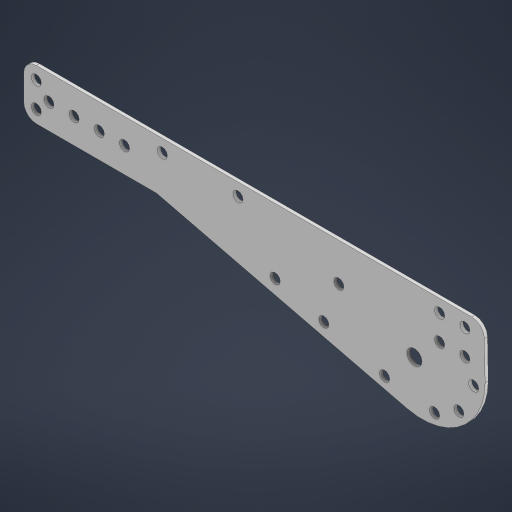
# Autodesk Inventor part: intake sled v5
Saved by Autodesk Inventor 2023.4 (Build 274418000, 418)
## iProperties
Created: 2023-12-16
Part Number: intake sled v5
Material: Generic
Document SubType Name: Modeling
Designer: Meer
Density: 1 g/cm^3
Appearance: Default
Author: Meer
Autodesk Inventor part; units mm, degrees
ref_plane "YZ Plane" through (0, 0, 0) normal (1, 0, 0) x (0, 1, 0)
ref_plane "XZ Plane" through (0, 0, 0) normal (0, 1, 0) x (-1, 0, 0)
ref_plane "XY Plane" through (0, 0, 0) normal (0, 0, 1) x (1, 0, 0)
sketch "Sketch1" plane through (0, 0, 0) normal (0, 0, 1) x (1, 0, 0)
  line L0 (0, 0) -> (247.65, 0)
  line L1 (247.65, 0) -> (247.65, 38.1)
  line L2 (247.65, 38.1) -> (0, 38.1)
  line L3 (0, 38.1) -> (0, 0)
  line L4 (286.1616, 0) -> (255.1962, 0)
  line L5 (255.1962, 0) -> (255.1962, 12.7)
  line L6 (255.1962, 12.7) -> (286.1616, 12.7)
  line L7 (286.1616, 12.7) -> (286.1616, 0)
  line L8 (247.65, 12.7) -> (200.66, 12.7)
  line L9 (16.2468, 38.1) -> (16.2468, 12.7)
  line L10 (16.2468, 12.7) -> (196.85, 12.7)
  line L11 (0, 12.7) -> (17.7951, 12.7)
  circle A0 centre (200.66, 12.7) radius 31.75
  line L12 (232.41, 12.7) -> (231.9451, 38.1)
  line L13 (66.8614, 12.7) -> (200.8653, -20.0324)
  line L14 (193.3963, -18.208) -> (168.91, 12.7)
  point P0 (187.853, -16.3524)
  point P1 (232.3887, 13.8619)
  point P2 (229.7594, 0)
  point P3 (181.61, 38.1)
  point P4 (219.71, 38.1)
  point P5 (171.5606, 0)
  dimension "d0" = 247.65
  dimension "d1" = 38.1
  dimension "d2" = 12.7
  dimension "d3" = 30.9654
  dimension "d4" = 46.99
  dimension "d10" = 25.4
  dimension "d54" = 63.5
  constraints: 30 end point, 10 point on line, 5 perpendicular, 4 parallel, 4 point on circle, 2 horizontal, 1 centre point, 1 coincident
  measures "d0" distance of L1.end L2.end
  measures "d1" distance of L0.end L1.end
  measures "d2" distance of L6.end L4.start
  measures "d3" distance of L5.end L6.end
  measures "d4" distance of L8.start L8.end
  measures "d10" distance of L9.start L9.end
  measures "d54" diameter of A0
extrude "Extrusion4" add sketch "Sketch1" along normal blind 1.5875 contours L13 L0 A0 | L13 L10 A0 L0 | L3 L2 L9 L11 | A0 L14 L0 | L0 L14 A0 | L10 L9 L2 A0 | L14 L0 A0 | L14 A0 L2 L12 L0 | L2 L12 A0
fillet "Fillet6" radius 6.35 3 edges at (0, 38.1, 0.7937) (0, 12.7, 0.7937) (231.9451, 38.1, 0.7937)
sketch "Sketch4" plane through (0, 0, 1.5875) normal (0, 0, 1) x (1, 0, 0)
  arc A0 (6.35, 38.1) -> (0, 31.75) centre (6.35, 31.75) ccw projected
  line L0 (6.35, 38.1) -> (6.35, 31.75)
  line L1 (6.35, 31.75) -> (0, 31.75)
  circle A1 centre (6.35, 31.75) radius 2.54
  line L2 (6.35, 31.75) -> (6.35, 19.05)
  circle A2 centre (6.35, 19.05) radius 2.54
  line L3 (6.35, 31.75) -> (57.15, 31.75)
  line L4 (57.15, 31.75) -> (107.95, 31.75)
  line L5 (107.95, 31.75) -> (158.75, 31.75)
  line L6 (158.75, 31.75) -> (209.55, 31.75)
  circle A3 centre (107.95, 31.75) radius 2.54
  circle A4 centre (209.55, 31.75) radius 2.54
  line L7 (57.15, 31.75) -> (57.15, 19.05)
  line L8 (57.15, 19.05) -> (107.95, 19.05)
  line L9 (107.95, 19.05) -> (158.75, 19.05)
  line L10 (158.75, 19.05) -> (209.55, 19.05)
  circle A5 centre (158.75, 19.05) radius 2.54
  circle A6 centre (209.55, 19.05) radius 2.54
  line L11 (225.7103, 38.1) -> (6.35, 38.1) projected
  arc A7 (193.3963, -18.208) -> (232.41, 12.7) centre (200.66, 12.7) ccw projected
  line L12 (209.55, 31.75) -> (196.85, 31.75)
  line L13 (196.85, 31.75) -> (196.85, 19.05)
  circle A8 centre (196.85, 31.75) radius 2.54
  line L14 (196.85, 19.05) -> (196.85, 6.096)
  circle A9 centre (196.85, 6.096) radius 3.81
  line L15 (57.15, 31.75) -> (69.85, 31.75)
  circle A10 centre (69.85, 31.75) radius 2.54
  point P0 (0, 0)
  point P1 (207.01, 31.75)
  dimension "d60" = 6.35
  dimension "d61" = 5.08
  dimension "d62" = 12.7
  dimension "d63" = 5.08
  dimension "d64" = 50.8
  dimension "d65" = 50.8
  dimension "d66" = 50.8
  dimension "d67" = 50.8
  dimension "d70" = 5.08
  dimension "d72" = 5.08
  dimension "d75" = 5.08
  dimension "d76" = 5.08
  dimension "d86" = 12.7
  dimension "d88" = 5.08
  dimension "d89" = 12.954
  dimension "d90" = 7.62
  dimension "d116" = 12.7
  dimension "d117" = 5.08
  constraints: 30 end point, 11 coincident, 9 centre point, 7 point on line, 5 perpendicular, 3 vertical, 1 horizontal
  measures "d60" distance of L0.start L0.end
  measures "d61" diameter of A1
  measures "d62" distance of L2.start L2.end
  measures "d63" diameter of A2
  measures "d64" distance of L2.start L3.end
  measures "d65" distance of L3.end L4.end
  measures "d66" distance of L4.end L5.end
  measures "d67" distance of L5.end L6.end
  measures "d70" diameter of A3
  measures "d72" diameter of A4
  measures "d75" diameter of A5
  measures "d76" diameter of A6
  measures "d86" distance of L12.start L12.end
  measures "d88" diameter of A8
  measures "d89" distance of L14.start L14.end
  measures "d90" diameter of A9
  measures "d116" distance of L7.start L15.end
  measures "d117" diameter of A10
extrude "Extrusion5" cut sketch "Sketch4" against normal blind 25.4 contours A1 L3 L0 | L0 L1 A1 | L1 L2 A1 | L3 A1 L2 | A2 | L4 A10 | L4 A10 | A3 L5 L4 | L4 L5 A3 | A5 L10 L9 | L9 L10 A5 | A4 | A6 | A9
sketch "Sketch5" plane through (0, 0, 1.5875) normal (0, 0, 1) x (1, 0, 0)
  circle A0 centre (209.55, 31.75) radius 2.54 projected
  line L0 (209.55, 31.75) -> (222.25, 31.75)
  line L1 (222.25, 31.75) -> (222.25, 19.05)
  line L2 (222.25, 19.05) -> (226.6625, 8.5061)
  line L3 (226.6625, 8.5061) -> (219.2036, -6.223)
  line L4 (219.2036, -6.223) -> (207.01, -13.0403)
  line L5 (207.01, -13.0403) -> (181.8398, -9.6316)
  line L6 (181.8398, -9.6316) -> (151.2071, -1.2828)
  line L7 (151.2071, -1.2828) -> (126.701, 5.3962)
  circle A1 centre (126.701, 5.3962) radius 2.54
  circle A2 centre (151.2071, -1.2828) radius 2.54
  circle A3 centre (181.8398, -9.6316) radius 2.54
  circle A4 centre (207.01, -13.0403) radius 2.54
  circle A5 centre (219.2036, -6.223) radius 2.54
  circle A6 centre (226.6625, 8.5061) radius 2.54
  circle A7 centre (222.25, 19.05) radius 2.54
  circle A8 centre (222.25, 31.75) radius 2.54
  circle A9 centre (6.35, 19.05) radius 2.54 projected
  line L8 (6.35, 19.05) -> (15.3303, 28.0303)
  line L9 (6.35, 19.05) -> (19.05, 19.05) construction
  circle A10 centre (6.35, 31.75) radius 2.54 projected
  line L10 (6.35, 31.75) -> (15.3303, 22.7697)
  line L11 (6.35, 31.75) -> (19.05, 31.75) construction
  circle A11 centre (12.7, 25.4) radius 2.54
  line L12 (12.7, 25.4) -> (50.8, 25.4)
  circle A12 centre (50.8, 25.4) radius 2.54
  line L13 (12.7, 25.4) -> (25.4, 25.4)
  line L14 (25.4, 25.4) -> (38.1, 25.4)
  circle A13 centre (25.4, 25.4) radius 2.54
  circle A14 centre (38.1, 25.4) radius 2.54
  point P0 (0, 0)
  dimension "d91" = 12.7
  dimension "d92" = 12.7
  dimension "d93" = 11.43
  dimension "d94" = 16.51
  dimension "d95" = 13.97
  dimension "d96" = 25.4
  dimension "d97" = 31.75
  dimension "d98" = 25.4
  dimension "d99" = 5.08
  dimension "d100" = 5.08
  dimension "d101" = 5.08
  dimension "d102" = 5.08
  dimension "d103" = 5.08
  dimension "d104" = 5.08
  dimension "d105" = 5.08
  dimension "d106" = 5.08
  dimension "d109" = 12.7
  dimension "d110" = 45
  dimension "d111" = 12.7
  dimension "d112" = 45
  dimension "d113" = 5.08
  dimension "d114" = 38.1
  dimension "d115" = 5.08
  dimension "d118" = 12.7
  dimension "d119" = 12.7
  dimension "d120" = 5.08
  dimension "d121" = 5.08
  constraints: 30 end point, 12 centre point, 11 coincident, 5 point on line, 4 horizontal, 2 equal length, 1 perpendicular
  measures "d91" distance of L0.start L0.end
  measures "d92" distance of L0.end L1.end
  measures "d93" distance of L1.end L2.end
  measures "d94" distance of L2.end L3.end
  measures "d95" distance of L3.end L4.end
  measures "d96" distance of L4.end L5.end
  measures "d97" distance of L5.end L6.end
  measures "d98" distance of L6.end L7.end
  measures "d99" diameter of A1
  measures "d100" diameter of A2
  measures "d101" diameter of A3
  measures "d102" diameter of A4
  measures "d103" diameter of A5
  measures "d104" diameter of A6
  measures "d105" diameter of A7
  measures "d106" diameter of A8
  measures "d109" distance of L8.start L8.end
  measures "d110" angle of L9 L8
  measures "d111" distance of L10.start L10.end
  measures "d112" angle of L10 L11
  measures "d113" diameter of A11
  measures "d114" distance of L12.start L12.end
  measures "d115" diameter of A12
  measures "d118" distance of L12.start L13.end
  measures "d119" distance of L13.end L14.end
  measures "d120" diameter of A13
  measures "d121" diameter of A14
extrude "Extrusion6" cut sketch "Sketch5" against normal blind 25.4 contours A8 L1 L0 | L0 L1 A8 | A7 L2 L1 | L1 L2 A7 | A6 L3 L2 | L2 L3 A6 | A5 L4 L3 | L3 L4 A5 | A4 L5 L4 | L4 L5 A4 | A3 L6 L5 | L5 L6 A3 | A2 L7 L6 | L6 L7 A2 | A1 | A11 L10 L8 | L8 L10 A11 | L10 A11 L8 | L12 A11 L10 | L8 A11 L12 | L12 A13 | L12 A13 | L12 A14 | L12 A14 | A12
body "Solid3"
